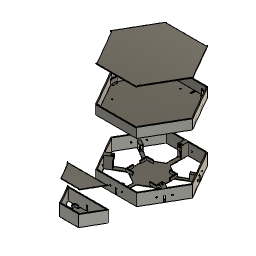
HiveLED (Autodesk Fusion 360 design; units mm, degrees)
Autodesk Fusion 360 part; units mm, degrees
sketch "Sketch1" plane through (0, 0, 0) normal (0, 0, 1) x (1, 0, 0) in component "base"
  line L0 (-43.3013, 75) -> (-86.6025, 0)
  line L1 (-86.6025, 0) -> (-43.3013, -75)
  line L2 (-43.3013, -75) -> (43.3013, -75)
  line L3 (43.3013, -75) -> (86.6025, 0)
  line L4 (86.6025, 0) -> (43.3013, 75)
  line L5 (43.3013, 75) -> (-43.3013, 75)
  line L6 (-84.2931, 0) -> (-42.1466, -73)
  line L7 (-42.1466, -73) -> (42.1466, -73)
  line L8 (42.1466, -73) -> (84.2931, 0)
  line L9 (84.2931, 0) -> (42.1466, 73)
  line L10 (42.1466, 73) -> (-42.1466, 73)
  line L11 (-42.1466, 73) -> (-84.2931, 0)
  dimension "d11" = 150
  dimension "d12" = -2
  constraint horizontal L3.end origin
  measures "d11" distance of L2 L5
extrude "Extrude11" add sketch "Sketch1" along normal blind 3 contours L0 L1 L2 L3 L4 L5 | L6 L7 L8 L9 L10 L11 makes body 1 in component "base"
extrude "Extrude12" add sketch "Sketch1" along normal blind 23 bodies 1 in component "base"
sketch "Sketch5" plane through (0, 0, 3) normal (0, 0, 1) x (-1, 0, 0)
  line L0 (84.2931, 0) -> (42.1466, 73)
  line L1 (42.1466, 73) -> (-42.1466, 73)
  line L2 (-42.1466, 73) -> (-84.2931, 0)
  line L3 (-84.2931, 0) -> (-42.1466, -73)
  line L4 (-42.1466, -73) -> (42.1466, -73)
  line L5 (42.1466, -73) -> (84.2931, 0)
  line L6 (79.53, -8.25) -> (79.53, 8.25)
  line L7 (46.9097, 64.75) -> (32.6203, 73)
  line L8 (-32.6203, 73) -> (-46.9097, 64.75)
  line L9 (-79.53, 8.25) -> (-79.53, -8.25)
  line L10 (-46.9097, -64.75) -> (-32.6203, -73)
  line L11 (32.6203, -73) -> (46.9097, -64.75)
  dimension "d82" = 16.5
  dimension "d84" = 360
  constraint coincident L5 L6.start
  constraint coincident L0 L6.end
  constraint vertical L6
  measures "d82" distance of L6.start L6.end
extrude "Extrude13" add sketch "Sketch5" along normal blind 10.1 contours L0 L5 L6 | L0 L1 L7 | L4 L5 L11 | L1 L2 L8 | L3 L4 L10 | L2 L3 L9 bodies 1 in component "base"
sketch "Sketch6" plane through (0, 0, 0) normal (0, 1, 0) x (1, 0, 0)
  line L0 (84.2931, -13.1) -> (84.2931, -23)
  line L1 (84.2931, -23) -> (86.6025, -23)
  line L2 (86.6025, -23) -> (86.6025, 0)
  line L3 (86.6025, 0) -> (-86.6025, 0)
  line L4 (-86.6025, 0) -> (-86.6025, -23)
  line L5 (-86.6025, -23) -> (-84.2931, -23)
  line L6 (-84.2931, -23) -> (-84.2931, -13.1)
  line L7 (-84.2931, -13.1) -> (-79.53, -13.1)
  line L8 (-79.53, -13.1) -> (-79.53, -3)
  line L9 (-79.53, -3) -> (79.53, -3)
  line L10 (79.53, -3) -> (79.53, -13.1)
  line L11 (79.53, -13.1) -> (84.2931, -13.1)
  line L12 (79.13, -3) -> (79.13, -5)
  line L13 (79.13, -5) -> (77.13, -3)
  dimension "d87" = 2
  dimension "d88" = 45
  dimension "d89" = 0.4
  constraint coincident L9 L12.start
  constraint perpendicular L9 L12
  constraint coincident L9 L13.end
  measures "d87" distance of L12.start L12.end
  measures "d88" angle of L12 L13
  measures "d89" distance of L10 L12
extrude "Extrude14" add sketch "Sketch6" along normal mid plane 10 contours L9 L12 L13 bodies 1 in component "base"
pattern_circular "C-Pattern3" count 6 over 360 about axis through (0, 0, 1.75) along (0, 0, 1) of "Extrude14" in component "base"
sketch "Sketch17" plane through (0, 0, 23) normal (0, 0, 1) x (-1, 0, 0) in component "base"
  line L0 (84.2931, 0) -> (42.1466, -73)
  line L1 (42.1466, -73) -> (-42.1466, -73)
  line L2 (-42.1466, -73) -> (-84.2931, 0)
  line L3 (-84.2931, 0) -> (-42.1466, 73)
  line L4 (-42.1466, 73) -> (42.1466, 73)
  line L5 (42.1466, 73) -> (84.2931, 0)
  line L6 (-43.3013, -75) -> (43.3013, -75)
  line L7 (43.3013, -75) -> (86.6025, 0)
  line L8 (86.6025, 0) -> (43.3013, 75)
  line L9 (43.3013, 75) -> (-43.3013, 75)
  line L10 (-43.3013, 75) -> (-86.6025, 0)
  line L11 (-86.6025, 0) -> (-43.3013, -75)
  line L12 (42.1466, 73) -> (43.3013, 75)
  line L13 (-43.3013, 75) -> (-42.1466, 73)
  line L14 (-42.1466, -73) -> (-43.3013, -75)
  line L15 (-84.2931, 0) -> (-86.6025, 0)
  line L16 (42.1466, -73) -> (43.3013, -75)
  line L17 (84.2931, 0) -> (86.6025, 0)
  constraint coincident L4.end L5.start
  constraint coincident L8.end L9.start
  constraint coincident L9.end L10.start
  constraint coincident L3.end L4.start
  constraint coincident L1.end L2.start
  constraint coincident L6.start L11.end
  constraint coincident L2.end L3.start
  constraint coincident L10.end L11.start
  constraint coincident L0.end L1.start
  constraint coincident L6.end L7.start
  constraint coincident L0.start L5.end
  constraint coincident L7.end L8.start
extrude "Extrude27" cut sketch "Sketch17" against normal blind 3 contours L0 L7 L16 L17 | L4 L9 L12 L13 | L2 L11 L14 L15 bodies 1 in component "base"
sketch "Sketch19" plane through (0, 0, 20) normal (0, 0, 1) x (-1, 0, 0) in component "base"
  line L0 (-43.3013, 75) -> (-42.1466, 73)
  line L1 (-42.1466, 73) -> (42.1466, 73)
  line L2 (42.1466, 73) -> (43.3013, 75)
  line L3 (43.3013, 75) -> (-43.3013, 75)
  line L4 (42.1466, -73) -> (43.3013, -75)
  line L5 (43.3013, -75) -> (86.6025, 0)
  line L6 (86.6025, 0) -> (84.2931, 0)
  line L7 (84.2931, 0) -> (42.1466, -73)
  line L8 (-42.1466, -73) -> (-84.2931, 0)
  line L9 (-84.2931, 0) -> (-86.6025, 0)
  line L10 (-86.6025, 0) -> (-43.3013, -75)
  line L11 (-43.3013, -75) -> (-42.1466, -73)
  line L12 (84.2931, 0) -> (42.1466, 73)
  line L13 (-42.1466, 73) -> (42.1466, 73)
  line L14 (-42.1466, 73) -> (-84.2931, 0)
  line L15 (-42.1466, -73) -> (42.1466, -73)
  constraint coincident L6.end L7.start
  constraint coincident L1.end L2.start
  constraint coincident L0.end L1.start
  constraint coincident L8.end L9.start
  constraint coincident L8.start L11.end
  constraint coincident L4.start L7.end
extrude "Extrude31" cut 1 faces at (14.4338, -25, 0) along direction (0, 0, 1) blind 1.3 on bodies 1 bodies 1 in component "base"
extrude "Extrude1" add sketch "Sketch19" along normal blind 3 separate body makes body 2 in component "Top"
sketch "Sketch23" plane through (0, 0, 3) normal (0, 0, 1) x (-1, 0, 0) in component "base"
  line L0 (-35.2349, 71.0286) -> (-34.2349, 69.2965)
  line L1 (-34.2349, 69.2965) -> (-42.8951, 64.2965)
  line L2 (-42.8951, 64.2965) -> (-43.8951, 66.0286)
  line L3 (-43.8951, 66.0286) -> (-35.2349, 71.0286)
  line L4 (43.8951, 66.0286) -> (42.8951, 64.2965)
  line L5 (42.8951, 64.2965) -> (34.2349, 69.2965)
  line L6 (34.2349, 69.2965) -> (35.2349, 71.0286)
  line L7 (35.2349, 71.0286) -> (43.8951, 66.0286)
  line L8 (79.13, -5) -> (77.13, -5)
  line L9 (77.13, -5) -> (77.13, 5)
  line L10 (77.13, 5) -> (79.13, 5)
  line L11 (79.13, 5) -> (79.13, -5)
  line L12 (35.2349, -71.0286) -> (34.2349, -69.2965)
  line L13 (34.2349, -69.2965) -> (42.8951, -64.2965)
  line L14 (42.8951, -64.2965) -> (43.8951, -66.0286)
  line L15 (43.8951, -66.0286) -> (35.2349, -71.0286)
  line L16 (-43.8951, -66.0286) -> (-42.8951, -64.2965)
  line L17 (-42.8951, -64.2965) -> (-34.2349, -69.2965)
  line L18 (-34.2349, -69.2965) -> (-35.2349, -71.0286)
  line L19 (-35.2349, -71.0286) -> (-43.8951, -66.0286)
  line L20 (-79.13, 5) -> (-77.13, 5)
  line L21 (-77.13, 5) -> (-77.13, -5)
  line L22 (-77.13, -5) -> (-79.13, -5)
  line L23 (-79.13, -5) -> (-79.13, 5)
  line L24 (46.9097, 64.75) -> (32.6203, 73)
  line L25 (32.6203, 73) -> (-32.6203, 73)
  line L26 (-32.6203, 73) -> (-46.9097, 64.75)
  line L27 (-46.9097, 64.75) -> (-79.53, 8.25)
  line L28 (-79.53, 8.25) -> (-79.53, -8.25)
  line L29 (-79.53, -8.25) -> (-46.9097, -64.75)
  line L30 (-46.9097, -64.75) -> (-32.6203, -73)
  line L31 (-32.6203, -73) -> (32.6203, -73)
  line L32 (32.6203, -73) -> (46.9097, -64.75)
  line L33 (46.9097, -64.75) -> (79.53, -8.25)
  line L34 (79.53, -8.25) -> (79.53, 8.25)
  line L35 (79.53, 8.25) -> (46.9097, 64.75)
  circle A0 centre (0, -61.45) radius 1.55
  point P0 (0, -61.45)
  dimension "d219" = 3.1
  dimension "d220" = 11.55
  constraint vertical origin A0.centre
  constraint coincident P0 A0.centre
  measures "d219" diameter of A0
  measures "d220" distance of L31 P0
extrude "Extrude38" cut sketch "Sketch23" against normal blind 1.7 contours A0 bodies 1 in component "base"
pattern_circular "C-Pattern5" count 3 over 360 about axis through (0, 0, 1.75) along (0, 0, 1) of "Extrude38" in component "base"
sketch "Sketch24" plane through (0, 0, 1.3) normal (0, 0, -1) x (1, 0, 0) in component "base"
  circle A0 centre (53.2173, 30.725) radius 1.55
  circle A1 centre (-53.2173, 30.725) radius 1.55
  circle A2 centre (0, -61.45) radius 1.55
  line L0 (-43.3013, -75) -> (43.3013, -75)
  line L1 (43.3013, -75) -> (86.6025, 0)
  line L2 (86.6025, 0) -> (43.3013, 75)
  line L3 (43.3013, 75) -> (-43.3013, 75)
  line L4 (-43.3013, 75) -> (-86.6025, 0)
  line L5 (-86.6025, 0) -> (-43.3013, -75)
  line L6 (-42.1466, -73) -> (42.1466, -73)
  line L7 (42.1466, -73) -> (84.2931, 0)
  line L8 (84.2931, 0) -> (42.1466, 73)
  line L9 (42.1466, 73) -> (-42.1466, 73)
  line L10 (-42.1466, 73) -> (-84.2931, 0)
  line L11 (-84.2931, 0) -> (-42.1466, -73)
  dimension "d230" = -2
extrude "Extrude1'" add sketch "Sketch24" along normal blind 25 separate body contours L0 L1 L2 L3 L4 L5 makes body 3 in component "Electronics Cabin"
sketch "Sketch1 (2)" plane through (64.9519, -37.5, 0) normal (0.866025, -0.5, 0) x (0.5, 0.866025, 0) in component "Electronics Cabin"
  line L0 (-43.3013, 1.3) -> (-43.3013, -23.7)
  line L1 (43.3013, -23.7) -> (43.3013, 1.3)
  line L2 (-1.5, -11.7) -> (1.5, -11.7)
  line L3 (1.5, -11.7) -> (1.5, -22.7)
  line L4 (1.5, -22.7) -> (-1.5, -22.7)
  line L5 (-1.5, -22.7) -> (-1.5, -11.7)
  line L6 (-1.5, -11.7) -> (1.5, -22.7) construction
  line L7 (1.5, -11.7) -> (-1.5, -22.7) construction
  line L8 (-42.1466, 1.3) -> (42.1466, 1.3) construction
  line L9 (42.1466, 1.3) -> (42.1466, -23.7) construction
  line L10 (42.1466, -23.7) -> (-42.1466, -23.7)
  line L11 (-42.1466, -23.7) -> (-42.1466, 1.3) construction
  line L12 (3, -24.2) -> (-3, -24.2)
  line L13 (-3, -24.2) -> (-3, -10.2)
  line L14 (-3, -10.2) -> (3, -10.2)
  line L15 (3, -10.2) -> (3, -24.2)
  point P0 (0, -17.2)
  dimension "d243" = 3
  dimension "d244" = 11
  dimension "d245" = 1
  dimension "d246" = -1.5
  constraint horizontal L2
  constraint perpendicular L2 L3
  constraint parallel L2 L4
  constraint parallel L3 L5
  constraint coincident L6 P0
  constraint coincident L7 P0
  constraint vertical origin P0
  measures "d243" distance of L3 L5
  measures "d244" distance of L2.end L3.end
  measures "d245" distance of L4 L10
extrude "Extrude2" add sketch "Sketch1 (2)" against normal blind 15.45 contours L10 L13 L14 L15 bodies 3 in component "Electronics Cabin"
extrude "Extrude4" cut sketch "Sketch1 (2)" against normal blind 2 contours L2 L3 L4 L5 bodies 3 in component "Electronics Cabin"
sketch "Sketch2" plane through (0, 0, -23.7) normal (0, 0, -1) x (1, 0, 0) in component "Electronics Cabin"
  line L0 (43.3013, 75) -> (-43.3013, 75)
  line L1 (-43.3013, 75) -> (-86.6025, 0)
  line L2 (-86.6025, 0) -> (-43.3013, -75)
  line L3 (-43.3013, -75) -> (43.3013, -75)
  line L4 (43.3013, -75) -> (86.6025, 0)
  line L5 (86.6025, 0) -> (43.3013, 75)
  line L6 (64.7199, 33.9019) -> (84.2931, 0)
  line L7 (84.2931, 0) -> (42.1466, -73)
  line L8 (42.1466, -73) -> (-42.1466, -73)
  line L9 (-42.1466, -73) -> (-84.2931, 0)
  line L10 (-84.2931, 0) -> (-42.1466, 73)
  line L11 (-42.1466, 73) -> (42.1466, 73)
  line L12 (61.7199, 39.0981) -> (50.0718, 32.3731)
  line L13 (53.0718, 27.1769) -> (64.7199, 33.9019)
  line L14 (42.1466, 73) -> (61.7199, 39.0981)
  line L15 (50.0718, 32.3731) -> (53.0718, 27.1769)
extrude "Extrude5" add sketch "Sketch2" against normal blind 1 contours L6 L7 L8 L9 L10 L11 L12 L13 L14 L15 bodies 3 in component "Electronics Cabin"
pattern_circular "C-Pattern1" count 6 over 360 about axis through (0, 0, 1.75) along (0, 0, 1) of "Extrude2", "Extrude4" in component "Electronics Cabin"
sketch "Sketch3" plane through (0, 0, 0) normal (1, 0, 0) x (0, 1, 0) in component "Electronics Cabin"
  line L0 (-75, -11.7) -> (-59.55, -11.7)
  line L1 (-59.55, -10.2) -> (-73, -10.2)
  line L2 (-73, -10.2) -> (-73, 1.3)
  line L3 (-73, 1.3) -> (-75, 1.3)
  line L4 (-75, 1.3) -> (-75, -11.7)
  line L5 (59.55, -11.7) -> (75, -11.7)
  line L6 (75, -11.7) -> (75, 1.3)
  line L7 (75, 1.3) -> (73, 1.3)
  line L8 (73, 1.3) -> (73, -10.2)
  line L9 (73, -10.2) -> (59.55, -10.2)
  line L10 (75, -22.7) -> (-75, -22.7)
  line L11 (-75, -22.7) -> (-75, -23.7)
  line L12 (-75, -23.7) -> (75, -23.7)
  line L13 (75, -23.7) -> (75, -22.7)
  line L14 (63, 3) -> (63, 1.3)
  line L15 (75, 1.3) -> (75, 23)
  line L16 (75, 23) -> (73, 23)
  line L17 (73, 23) -> (73, 3)
  line L18 (59.9, 1.3) -> (59.9, 3)
  line L19 (63, 1.3) -> (75, 1.3)
  line L20 (-73, 20) -> (-75, 20)
  line L21 (-75, 20) -> (-75, 1.3)
  line L22 (-75, 1.3) -> (59.9, 1.3)
  line L23 (73, 3) -> (63, 3)
  line L24 (59.9, 3) -> (-73, 3)
  line L25 (-73, 3) -> (-73, 20)
  line L26 (58.65, 1.3) -> (58.65, -3.6)
  line L27 (58.65, -0.2) -> (64.25, -0.2)
  line L28 (64.25, -0.2) -> (64.25, -2.6)
  line L29 (64.25, -2.6) -> (58.65, -2.6)
  line L30 (61.45, -0.2) -> (61.45, -2.6) construction
  line L31 (59.9, 3) -> (63, 3) construction
  line L32 (59.55, -10.2) -> (58.65, -3.6)
  line L33 (59.55, -10.2) -> (58.5867, -10.2117) construction
  line L34 (75, 1.3) -> (63, 1.3)
  line L35 (-59.55, -11.7) -> (-59.55, -10.2)
  line L36 (59.55, -10.2) -> (59.55, -11.7)
  line L37 (59.9, 1.3) -> (63, 1.3)
  point P0 (61.45, 3)
  dimension "d255" = 5.6
  dimension "d256" = 1.5
  dimension "d258" = 2.4
  dimension "d260" = 1
  constraint coincident L19 L26.start
  constraint perpendicular L19 L26
  constraint coincident L26 L27.start
  constraint perpendicular L26 L27
  constraint perpendicular L27 L28
  constraint coincident L26 L29.end
  constraint perpendicular L26 L29
  constraint midpoint L27 L30.start
  constraint midpoint L29 L30.end
  constraint coincident L18.end L24.start
  constraint coincident L14.start L23.end
  constraint midpoint L31 P0
  constraint vertical L30.start P0
  constraint coincident L9.end L32.start
  constraint coincident L6.end L7.start
  constraint coincident L14.end L19.start
  constraint coincident L18.start L22.end
  measures "d255" distance of L27.start L27.end
  measures "d256" distance of L19 L27
  measures "d258" distance of L27 L29
  measures "d260" distance of L26.end L29.end
extrude "Extrude6" add sketch "Sketch3" along normal mid plane 8.2 contours L8 L9 L19 L22 L26 L27 L28 L29 L32 L34 L37 bodies 3 in component "Electronics Cabin"
sketch "Sketch4" plane through (0, 58.65, 0) normal (0, -1, 0) x (1, 0, 0) in component "Electronics Cabin"
  line L0 (-4.1, -3.6) -> (4.1, -3.6)
  line L1 (4.1, -3.6) -> (4.1, -2.6)
  line L2 (4.1, -2.6) -> (-4.1, -2.6)
  line L3 (-4.1, -2.6) -> (-4.1, -3.6)
  line L4 (-4.1, -0.2) -> (4.1, -0.2)
  line L5 (4.1, -0.2) -> (4.1, 1.3)
  line L6 (-4.1, 1.3) -> (-4.1, -0.2)
  line L7 (-4.1, -0.2) -> (-2.8, -0.2)
  line L8 (-2.8, -0.2) -> (-2.8, -2.6)
  line L9 (-2.8, -2.6) -> (-4.1, -2.6)
  line L10 (-4.1, -2.6) -> (-4.1, -0.2)
  line L11 (4.1, -0.2) -> (2.8, -0.2)
  line L12 (2.8, -0.2) -> (2.8, -2.6)
  line L13 (2.8, -2.6) -> (4.1, -2.6)
  line L14 (4.1, -2.6) -> (4.1, -0.2)
  line L15 (4.1, 1.3) -> (-4.1, 1.3)
  dimension "d287" = 5.6
  constraint horizontal L7
  constraint vertical L8
  constraint horizontal L9
  constraint vertical L10
  constraint coincident L2 L8.end
  constraint coincident L4.start L6.end
  constraint horizontal L11
  constraint vertical L12
  constraint horizontal L13
  constraint vertical L14
  constraint coincident L2 L12.end
  constraint coincident L4.end L5.start
  constraint equal L7 L11
  measures "d287" distance of L8 L12
extrude "Extrude7" add sketch "Sketch4" against normal blind 5.6 contours L2 L4 L7 L8 L9 L10 | L2 L4 L11 L12 L13 L14 bodies 3 in component "Electronics Cabin"
sketch "Sketch5 (2)" plane through (0, 0, 1.3) normal (0, 0, 1) x (-1, 0, 0) in component "Electronics Cabin"
  line L0 (84.2931, 0) -> (42.1466, -73)
  line L1 (42.1466, -73) -> (4.1, -73)
  line L2 (-42.1466, -73) -> (-84.2931, 0)
  line L3 (-84.2931, 0) -> (-42.1466, 73)
  line L4 (-42.1466, 73) -> (42.1466, 73)
  line L5 (42.1466, 73) -> (84.2931, 0)
  line L6 (43.3013, -75) -> (86.6025, 0)
  line L7 (86.6025, 0) -> (43.3013, 75)
  line L8 (43.3013, 75) -> (-43.3013, 75)
  line L9 (-43.3013, 75) -> (-86.6025, 0)
  line L10 (-86.6025, 0) -> (-43.3013, -75)
  line L11 (-43.3013, -75) -> (43.3013, -75)
  circle A0 centre (0, -61.45) radius 1.55
  line L12 (4.1, -73) -> (4.1, -58.65)
  line L13 (4.1, -58.65) -> (-4.1, -58.65)
  line L14 (-4.1, -58.65) -> (-4.1, -73)
  line L15 (-4.1, -73) -> (-42.1466, -73)
extrude "Extrude9" cut sketch "Sketch5 (2)" against normal blind 9 contours A0 bodies 3 in component "Electronics Cabin"
sketch "Sketch6 (2)" plane through (0, 0, -0.2) normal (0, 0, -1) x (1, 0, 0) in component "Electronics Cabin"
  circle A0 centre (0, -61.45) radius 1.55
  line L0 (2.8, -58.65) -> (-2.8, -58.65)
  line L1 (-2.8, -64.25) -> (2.8, -64.25)
  circle A1 centre (0, -61.45) radius 1.55
  line L2 (2.8, -64.25) -> (2.8, -58.65)
  line L3 (-2.8, -58.65) -> (-2.8, -64.25)
extrude "Extrude10" add sketch "Sketch6 (2)" against normal blind 0.3 contours A0 A1 bodies 3 in component "Electronics Cabin"
extrude "Extrude14'" add 2 faces at (-3.3667, 68.5167, -10.2) (3.3667, 64.0333, -10.2) along direction (0, 0, -1) blind 12.7 on bodies 3 bodies 3 in component "Electronics Cabin"
pattern_circular "C-Pattern2" count 3 over 360 about axis through (0, 0, 1.75) along (0, 0, 1) of "Extrude6", "Extrude7", "Extrude9", "Extrude10", "Extrude14'" in component "Electronics Cabin"
sketch "Sketch9" plane through (0, 0, 3) normal (0, 0, 1) x (-1, 0, 0)
  line L0 (-35.2349, 71.0286) -> (-34.2349, 69.2965)
  line L1 (-34.2349, 69.2965) -> (-42.8951, 64.2965)
  line L2 (-42.8951, 64.2965) -> (-43.8951, 66.0286)
  line L3 (-43.8951, 66.0286) -> (-35.2349, 71.0286)
  line L4 (43.8951, 66.0286) -> (42.8951, 64.2965)
  line L5 (42.8951, 64.2965) -> (34.2349, 69.2965)
  line L6 (34.2349, 69.2965) -> (35.2349, 71.0286)
  line L7 (35.2349, 71.0286) -> (43.8951, 66.0286)
  line L8 (79.13, -5) -> (77.13, -5)
  line L9 (77.13, -5) -> (77.13, 5)
  line L10 (77.13, 5) -> (79.13, 5)
  line L11 (79.13, 5) -> (79.13, -5)
  line L12 (35.2349, -71.0286) -> (34.2349, -69.2965)
  line L13 (34.2349, -69.2965) -> (42.8951, -64.2965)
  line L14 (42.8951, -64.2965) -> (43.8951, -66.0286)
  line L15 (43.8951, -66.0286) -> (35.2349, -71.0286)
  line L16 (-43.8951, -66.0286) -> (-42.8951, -64.2965)
  line L17 (-42.8951, -64.2965) -> (-34.2349, -69.2965)
  line L18 (-34.2349, -69.2965) -> (-35.2349, -71.0286)
  line L19 (-35.2349, -71.0286) -> (-43.8951, -66.0286)
  line L20 (-79.13, 5) -> (-77.13, 5)
  line L21 (-77.13, 5) -> (-77.13, -5)
  line L22 (-77.13, -5) -> (-79.13, -5)
  line L23 (-79.13, -5) -> (-79.13, 5)
  line L24 (46.9097, 64.75) -> (32.6203, 73)
  line L25 (32.6203, 73) -> (-32.6203, 73)
  line L26 (-32.6203, 73) -> (-46.9097, 64.75)
  line L27 (-46.9097, 64.75) -> (-79.53, 8.25)
  line L28 (-79.53, 8.25) -> (-79.53, -8.25)
  line L29 (-79.53, -8.25) -> (-46.9097, -64.75)
  line L30 (-46.9097, -64.75) -> (-32.6203, -73)
  line L31 (-32.6203, -73) -> (32.6203, -73)
  line L32 (32.6203, -73) -> (46.9097, -64.75)
  line L33 (46.9097, -64.75) -> (79.53, -8.25)
  line L34 (79.53, -8.25) -> (79.53, 8.25)
  line L35 (79.53, 8.25) -> (46.9097, 64.75)
  line L36 (-17.6203, -63.5) -> (-20.6203, -63.5)
  line L37 (-20.6203, -63.5) -> (-20.6203, -71.5)
  line L38 (-20.6203, -71.5) -> (-17.6203, -71.5)
  line L39 (-17.6203, -71.5) -> (-17.6203, -63.5)
  line L40 (-17.6203, -63.5) -> (-20.6203, -71.5) construction
  line L41 (-20.6203, -63.5) -> (-17.6203, -71.5) construction
  circle A0 centre (-53.2173, 30.725) radius 1.55
  circle A1 centre (53.2173, 30.725) radius 1.55
  circle A2 centre (0, -61.45) radius 1.55
  point P0 (-19.1203, -67.5)
  dimension "d319" = 8
  dimension "d320" = 3
  dimension "d321" = 1.5
  dimension "d322" = 12
  constraint horizontal L36
  constraint perpendicular L36 L37
  constraint parallel L36 L38
  constraint parallel L37 L39
  constraint coincident L40 P0
  constraint coincident L41 P0
  measures "d319" distance of L36.end L37.end
  measures "d320" distance of L37.end L38.end
  measures "d321" distance of L31 L38
  measures "d322" distance of L30.end L37
extrude "Extrude40" cut sketch "Sketch9" against normal blind 1.7 contours L36 L37 L38 L39 bodies 1 in component "base"
extrude "Extrude41" cut 3 faces at (14.0489, 74.3333, 23) (-71.399, -25, 23) (57.3501, -49.3333, 23) along direction (0, 0, -1) blind 1.3 on bodies 1 bodies 1 in component "base"
sketch "Sketch7" plane through (0, 0, -23.7) normal (0, 0, -1) x (1, 0, 0) in component "Electronics Cabin"
  line L0 (43.3013, 75) -> (-43.3013, 75)
  line L1 (-43.3013, 75) -> (-86.6025, 0)
  line L2 (-86.6025, 0) -> (-43.3013, -75)
  line L3 (-43.3013, -75) -> (43.3013, -75)
  line L4 (43.3013, -75) -> (86.6025, 0)
  line L5 (86.6025, 0) -> (43.3013, 75)
  line L6 (52.3218, -28.476) -> (65.7019, -36.201)
  line L7 (65.7019, -36.201) -> (64.2019, -38.799)
  line L8 (64.2019, -38.799) -> (50.8218, -31.074)
  line L9 (53.0718, -27.1769) -> (52.3218, -28.476)
  line L10 (84.2931, 0) -> (64.7199, -33.9019)
  line L11 (42.1466, -73) -> (4.1, -73)
  line L12 (1.5, -59.55) -> (1.5, -75)
  line L13 (1.5, -75) -> (-1.5, -75)
  line L14 (-1.5, -75) -> (-1.5, -59.55)
  line L15 (4.1, -59.55) -> (1.5, -59.55)
  line L16 (-4.1, -73) -> (-42.1466, -73)
  line L17 (-42.1466, -73) -> (-61.7199, -39.0981)
  line L18 (-50.8218, -31.074) -> (-64.2019, -38.799)
  line L19 (-64.2019, -38.799) -> (-65.7019, -36.201)
  line L20 (-65.7019, -36.201) -> (-52.3218, -28.476)
  line L21 (-50.0718, -32.3731) -> (-50.8218, -31.074)
  line L22 (-64.7199, -33.9019) -> (-84.2931, 0)
  line L23 (-84.2931, 0) -> (-65.2699, 32.9493)
  line L24 (-52.3218, 28.476) -> (-65.7019, 36.201)
  line L25 (-65.7019, 36.201) -> (-64.2019, 38.799)
  line L26 (-64.2019, 38.799) -> (-50.8218, 31.074)
  line L27 (-53.6218, 26.2243) -> (-52.3218, 28.476)
  line L28 (-61.1699, 40.0507) -> (-42.1466, 73)
  line L29 (-42.1466, 73) -> (-3, 73)
  line L30 (-1.5, 59.55) -> (-1.5, 75)
  line L31 (-1.5, 75) -> (1.5, 75)
  line L32 (1.5, 75) -> (1.5, 59.55)
  line L33 (-3, 59.55) -> (-1.5, 59.55)
  line L34 (3, 73) -> (42.1466, 73)
  line L35 (42.1466, 73) -> (61.1699, 40.0507)
  line L36 (50.8218, 31.074) -> (64.2019, 38.799)
  line L37 (64.2019, 38.799) -> (65.7019, 36.201)
  line L38 (65.7019, 36.201) -> (52.3218, 28.476)
  line L39 (65.2699, 32.9493) -> (84.2931, 0)
  line L40 (49.5218, 33.3257) -> (50.8218, 31.074)
  line L41 (0, 37.5278) -> (-32.5, 18.7639)
  line L42 (-32.5, 18.7639) -> (-32.5, -18.7639)
  line L43 (-32.5, -18.7639) -> (0, -37.5278)
  line L44 (0, -37.5278) -> (32.5, -18.7639)
  line L45 (32.5, -18.7639) -> (32.5, 18.7639)
  line L46 (32.5, 18.7639) -> (0, 37.5278)
  line L47 (4.1, -73) -> (4.1, -59.55)
  line L48 (-1.5, -59.55) -> (-4.1, -59.55)
  line L49 (-4.1, -59.55) -> (-4.1, -73)
  line L50 (-65.2699, 32.9493) -> (-53.6218, 26.2243)
  line L51 (-49.5218, 33.3257) -> (-61.1699, 40.0507)
  line L52 (61.1699, 40.0507) -> (49.5218, 33.3257)
  line L53 (52.3218, 28.476) -> (53.6218, 26.2243)
  line L54 (53.6218, 26.2243) -> (65.2699, 32.9493)
  line L55 (64.7199, -33.9019) -> (53.0718, -27.1769)
  line L56 (50.8218, -31.074) -> (50.0718, -32.3731)
  line L57 (50.0718, -32.3731) -> (61.7199, -39.0981)
  line L58 (61.7199, -39.0981) -> (42.1466, -73)
  line L59 (-61.7199, -39.0981) -> (-50.0718, -32.3731)
  line L60 (-52.3218, -28.476) -> (-53.0718, -27.1769)
  line L61 (-53.0718, -27.1769) -> (-64.7199, -33.9019)
  line L62 (-50.8218, 31.074) -> (-49.5218, 33.3257)
  line L63 (-3, 73) -> (-3, 59.55)
  line L64 (1.5, 59.55) -> (3, 59.55)
  line L65 (3, 59.55) -> (3, 73)
  line L66 (-4.1, -59.55) -> (-4.1, -35.1606)
  line L67 (4.1, -59.55) -> (4.1, -35.1606)
  line L68 (53.6218, 26.2243) -> (32.5, 14.0296)
  line L69 (49.5218, 33.3257) -> (28.4, 21.131)
  line L70 (-49.5218, 33.3257) -> (-28.4, 21.131)
  line L71 (-53.6218, 26.2243) -> (-32.5, 14.0296)
  line L72 (-50.0718, -32.3731) -> (-29.5, -20.4959)
  line L73 (-53.0718, -27.1769) -> (-32.5, -15.2998)
  line L74 (50.0718, -32.3731) -> (29.5, -20.4959)
  line L75 (53.0718, -27.1769) -> (32.5, -15.2998)
  line L76 (3, 59.55) -> (3, 35.7957)
  line L77 (-3, 59.55) -> (-3, 35.7957)
  dimension "d288" = 65
  dimension "d361" = 360
  dimension "d363" = 360
  constraint vertical L41.start origin
  constraint coincident L48.end L49.start
  constraint coincident L43 L66.end
  constraint perpendicular L48 L66
  constraint coincident L15.start L47.end
  constraint coincident L44 L67.end
  constraint perpendicular L15 L67
  constraint coincident L21.start L59.end
  constraint coincident L43 L72.end
  constraint perpendicular L21 L72
  constraint coincident L60.end L61.start
  constraint coincident L42 L73.end
  constraint perpendicular L60 L73
  measures "d288" distance of L42 L45
extrude "Extrude12'" cut sketch "Sketch7" against normal blind 1 contours L34 L35 L46 L52 L65 L69 L76 | L28 L29 L41 L51 L63 L70 L77 | L10 L39 L45 L54 L55 L68 L75 | L22 L23 L42 L50 L61 L71 L73 | L11 L44 L47 L57 L58 L67 L74 | L16 L17 L43 L49 L59 L66 L72 bodies 3 in component "Electronics Cabin"
sketch "Sketch8" plane through (0, 0, -22.7) normal (0, 0, 1) x (-1, 0, 0) in component "Electronics Cabin"
  line L0 (-29.5, -20.4959) -> (-4.1, -35.1606)
  line L1 (4.1, -35.1606) -> (29.5, -20.4959)
  line L2 (32.5, -15.2998) -> (32.5, 14.0296)
  line L3 (28.4, 21.131) -> (3, 35.7957)
  line L4 (-3, 35.7957) -> (-28.4, 21.131)
  line L5 (-32.5, 14.0296) -> (-32.5, -15.2998)
  line L6 (30.5, -20.5) -> (-30.5, -20.5)
  line L7 (-30.5, -20.5) -> (-30.5, 20.5)
  line L8 (-30.5, 20.5) -> (30.5, 20.5)
  line L9 (30.5, 20.5) -> (30.5, -20.5)
  line L10 (30.5, -20.5) -> (-30.5, 20.5) construction
  line L11 (-30.5, -20.5) -> (30.5, 20.5) construction
  line L12 (-32.5, 22.5) -> (32.5, 22.5)
  line L13 (32.5, 22.5) -> (32.5, -22.5)
  line L14 (32.5, -22.5) -> (-32.5, -22.5)
  line L15 (-32.5, -22.5) -> (-32.5, 22.5)
  line L16 (17.5, -22.5) -> (17.5, -20.5)
  line L17 (32.5, -7.5) -> (30.5, -7.5)
  line L18 (-20, 0) -> (-2.5, 0)
  line L19 (32.5, 7.5) -> (30.5, 7.5)
  line L20 (17.5, 22.5) -> (17.5, 20.5)
  line L21 (0, -2.5) -> (0, -20)
  line L22 (-17.5, -22.5) -> (-17.5, -20.5)
  line L23 (-32.5, -7.5) -> (-30.5, -7.5)
  line L24 (-32.5, 7.5) -> (-30.5, 7.5)
  line L25 (-17.5, 22.5) -> (-17.5, 20.5)
  line L26 (-32.5, 14.0296) -> (-32.5, -15.2998)
  line L27 (-29.5, -20.4959) -> (-4.1, -35.1606)
  line L28 (4.1, -35.1606) -> (29.5, -20.4959)
  line L29 (32.5, -15.2998) -> (32.5, 14.0296)
  line L30 (28.4, 21.131) -> (3, 35.7957)
  line L31 (-3, 35.7957) -> (-28.4, 21.131)
  line L32 (-4.1, -35.1606) -> (-4.1, -59.55)
  line L33 (-4.1, -59.55) -> (-1.5, -59.55)
  line L34 (-1.5, -59.55) -> (-1.5, -75)
  line L35 (-1.5, -75) -> (1.5, -75)
  line L36 (4.1, -59.55) -> (4.1, -35.1606)
  line L37 (-28.4, 21.131) -> (-49.5218, 33.3257)
  line L38 (53.6218, 26.2243) -> (52.3218, 28.476)
  line L39 (52.3218, 28.476) -> (65.7019, 36.201)
  line L40 (65.7019, 36.201) -> (64.2019, 38.799)
  line L41 (-53.6218, 26.2243) -> (-32.5, 14.0296)
  line L42 (-50.8218, 31.074) -> (-64.2019, 38.799)
  line L43 (-64.2019, 38.799) -> (-65.7019, 36.201)
  line L44 (-4.1, -35.1606) -> (-4.1, -59.55)
  line L45 (-4.1, -59.55) -> (-1.5, -59.55)
  line L46 (-1.5, -59.55) -> (-1.5, -75)
  line L47 (-1.5, -75) -> (1.5, -75)
  line L48 (4.1, -59.55) -> (4.1, -35.1606)
  line L49 (-28.4, 21.131) -> (-49.5218, 33.3257)
  line L50 (53.6218, 26.2243) -> (52.3218, 28.476)
  line L51 (52.3218, 28.476) -> (65.7019, 36.201)
  line L52 (65.7019, 36.201) -> (64.2019, 38.799)
  line L53 (-53.6218, 26.2243) -> (-32.5, 14.0296)
  line L54 (-50.8218, 31.074) -> (-64.2019, 38.799)
  line L55 (-64.2019, 38.799) -> (-65.7019, 36.201)
  line L56 (-32.5, -15.2998) -> (-53.0718, -27.1769)
  line L57 (-53.0718, -27.1769) -> (-52.3218, -28.476)
  line L58 (-52.3218, -28.476) -> (-65.7019, -36.201)
  line L59 (-65.7019, -36.201) -> (-64.2019, -38.799)
  line L60 (-64.2019, -38.799) -> (-50.8218, -31.074)
  line L61 (-50.8218, -31.074) -> (-50.0718, -32.3731)
  line L62 (-50.0718, -32.3731) -> (-29.5, -20.4959)
  line L63 (1.5, -75) -> (1.5, -59.55)
  line L64 (1.5, -59.55) -> (4.1, -59.55)
  line L65 (29.5, -20.4959) -> (50.0718, -32.3731)
  line L66 (50.0718, -32.3731) -> (50.8218, -31.074)
  line L67 (50.8218, -31.074) -> (64.2019, -38.799)
  line L68 (64.2019, -38.799) -> (65.7019, -36.201)
  line L69 (65.7019, -36.201) -> (52.3218, -28.476)
  line L70 (52.3218, -28.476) -> (53.0718, -27.1769)
  line L71 (53.0718, -27.1769) -> (32.5, -15.2998)
  line L72 (32.5, 14.0296) -> (53.6218, 26.2243)
  line L73 (64.2019, 38.799) -> (50.8218, 31.074)
  line L74 (50.8218, 31.074) -> (49.5218, 33.3257)
  line L75 (49.5218, 33.3257) -> (28.4, 21.131)
  line L76 (3, 35.7957) -> (3, 59.55)
  line L77 (3, 59.55) -> (1.5, 59.55)
  line L78 (1.5, 59.55) -> (1.5, 75)
  line L79 (1.5, 75) -> (-1.5, 75)
  line L80 (-1.5, 75) -> (-1.5, 59.55)
  line L81 (-1.5, 59.55) -> (-3, 59.55)
  line L82 (-3, 59.55) -> (-3, 35.7957)
  line L83 (-49.5218, 33.3257) -> (-50.8218, 31.074)
  line L84 (-65.7019, 36.201) -> (-52.3218, 28.476)
  line L85 (-52.3218, 28.476) -> (-53.6218, 26.2243)
  line L86 (-32.5, -15.2998) -> (-53.0718, -27.1769)
  line L87 (-53.0718, -27.1769) -> (-52.3218, -28.476)
  line L88 (-52.3218, -28.476) -> (-65.7019, -36.201)
  line L89 (-65.7019, -36.201) -> (-64.2019, -38.799)
  line L90 (-64.2019, -38.799) -> (-50.8218, -31.074)
  line L91 (-50.8218, -31.074) -> (-50.0718, -32.3731)
  line L92 (-50.0718, -32.3731) -> (-29.5, -20.4959)
  line L93 (1.5, -75) -> (1.5, -59.55)
  line L94 (1.5, -59.55) -> (4.1, -59.55)
  line L95 (29.5, -20.4959) -> (50.0718, -32.3731)
  line L96 (50.0718, -32.3731) -> (50.8218, -31.074)
  line L97 (50.8218, -31.074) -> (64.2019, -38.799)
  line L98 (64.2019, -38.799) -> (65.7019, -36.201)
  line L99 (65.7019, -36.201) -> (52.3218, -28.476)
  line L100 (52.3218, -28.476) -> (53.0718, -27.1769)
  line L101 (53.0718, -27.1769) -> (32.5, -15.2998)
  line L102 (32.5, 14.0296) -> (53.6218, 26.2243)
  line L103 (64.2019, 38.799) -> (50.8218, 31.074)
  line L104 (50.8218, 31.074) -> (49.5218, 33.3257)
  line L105 (49.5218, 33.3257) -> (28.4, 21.131)
  line L106 (3, 35.7957) -> (3, 59.55)
  line L107 (3, 59.55) -> (1.5, 59.55)
  line L108 (1.5, 59.55) -> (1.5, 75)
  line L109 (1.5, 75) -> (-1.5, 75)
  line L110 (-1.5, 75) -> (-1.5, 59.55)
  line L111 (-1.5, 59.55) -> (-3, 59.55)
  line L112 (-3, 59.55) -> (-3, 35.7957)
  line L113 (-49.5218, 33.3257) -> (-50.8218, 31.074)
  line L114 (-65.7019, 36.201) -> (-52.3218, 28.476)
  line L115 (-52.3218, 28.476) -> (-53.6218, 26.2243)
  dimension "d293" = 61
  dimension "d294" = 41
  dimension "d295" = -2
  dimension "d298" = 15
  dimension "d299" = 15
  constraint horizontal L6
  constraint perpendicular L6 L7
  constraint parallel L6 L8
  constraint parallel L7 L9
  constraint coincident L10 origin
  constraint coincident L11 origin
  constraint coincident L14 L16.start
  constraint coincident L6 L16.end
  constraint perpendicular L6 L16
  constraint coincident L2 L17.start
  constraint coincident L9 L17.end
  constraint perpendicular L9 L17
  constraint symmetric L16.start L18 L20.start
  constraint symmetric L16.end L18 L20.end
  constraint symmetric L17.start L18 L19.start
  constraint symmetric L17.end L18 L19.end
  constraint symmetric L16.start L21 L22.start
  constraint symmetric L16.end L21 L22.end
  constraint symmetric L17.start L21 L23.start
  constraint symmetric L17.end L21 L23.end
  constraint symmetric L19.start L21 L24.start
  constraint symmetric L19.end L21 L24.end
  constraint symmetric L20.start L21 L25.start
  constraint symmetric L20.end L21 L25.end
  measures "d293" distance of L7.end L8.end
  measures "d294" distance of L6.end L7.end
  measures "d298" distance of L13 L16
  measures "d299" distance of L14 L17
extrude "Extrude13'" add sketch "Sketch8" along normal blind 5 contours L0 L6 L14 L22 L27 | L0 L6 L14 L15 L27 L62 L92 | L5 L6 L7 L15 L23 L26 L62 L92 | L1 L6 L14 L16 L28 | L1 L6 L13 L14 L28 L65 L95 | L4 L5 L7 L8 L12 L15 L24 L25 L26 L31 L37 L49 | L2 L6 L9 L13 L17 L29 L65 L95 | L2 L3 L8 L9 L12 L13 L19 L20 L29 L30 L75 L105 | L4 L12 L31 L37 L49 | L3 L12 L30 L75 L105 bodies 3 in component "Electronics Cabin"
extrude "Extrude15" add 4 faces at (29.3406, 21.8333, -22.7) (-29.3406, 21.8333, -22.7) (-28.4, -22.0437, -22.7) (28.4, -22.0437, -22.7) along direction (0, 0, -1) blind 1 on bodies 3 bodies 3 in component "Electronics Cabin"
extrude "Extrude2'" cut 1 faces at (14.0489, -24.3333, 23) along direction (0, 0, -1) blind 1.3 on bodies 2 bodies 2 in component "Top"
extrude "Extrude42" add 6 faces at (-40.5589, 70.25, 13.1) (40.5589, 70.25, 13.1) (81.1177, 0, 13.1) (40.5589, -70.25, 13.1) (-40.5589, -70.25, 13.1) (-81.1177, 0, 13.1) along direction (0, 0, 1) blind 1 on bodies 1 bodies 1 in component "base"
sketch "Sketch26" plane through (0, 0, 14.1) normal (0, 0, 1) x (-1, 0, 0) in component "base"
  line L0 (42.1466, -73) -> (46.9097, -64.75)
  line L1 (46.9097, -64.75) -> (32.6203, -73)
  line L2 (32.6203, -73) -> (42.1466, -73)
  line L3 (45.9097, -66.4821) -> (34.6203, -73)
  line L4 (46.6499, -64.9) -> (56.8868, -47.1692)
  line L5 (56.8868, -47.1692) -> (12.4064, -72.85)
  line L6 (12.4064, -72.85) -> (32.8801, -72.85)
  line L7 (42.1466, -73) -> (84.2931, 0)
  line L8 (45.6499, -66.6321) -> (42.06, -72.85)
  line L9 (42.06, -72.85) -> (34.8801, -72.85)
  line L10 (34.8801, -72.85) -> (32.8801, -72.85)
  line L11 (45.6499, -66.6321) -> (46.6499, -64.9)
  dimension "d364" = 1
  dimension "d365" = 0.15
  dimension "d366" = 0.15
  dimension "d367" = 15
  dimension "d368" = 0.15
  dimension "d369" = 0.15
  constraint coincident L0 L3.start
  constraint coincident L2 L3.end
  constraint parallel L1 L3
  constraint coincident L1 L4.start
  constraint coincident L1 L6.end
  constraint horizontal L6
  constraint parallel L4 L7
  constraint parallel L1 L5
  constraint coincident L3 L8.start
  constraint coincident L3 L9.end
  constraint horizontal L9
  constraint parallel L7 L8
  measures "d364" distance of L1 L3
  measures "d365" distance of L4 L7
  measures "d366" distance of L2 L6
  measures "d367" distance of L0.start L5
  measures "d368" distance of L0 L8
  measures "d369" distance of L2 L9
extrude "Extrude43" cut sketch "Sketch26" against normal blind 2 contours L0 L2 L3 L7 L8 L9 | L3 L8 L9 bodies 1 in component "base"
pattern_circular "C-Pattern6" count 6 over 360 about axis through (0, 0, 1.75) along (0, 0, 1) of "Extrude43" in component "base"
extrude "Extrude44" add sketch "Sketch26" against normal blind 2 separate body contours L3 L8 L9 makes body 4 in component "base"
extrude "Extrude45" add sketch "Sketch26" along normal blind 1 separate body contours L3 L8 L9 | L1 L3 L10 L11 | L1 L4 L5 L6 makes body 5 in component "base"
combine "Combine4" operation add target body 5 tool bodies 4 in component "base"
sketch "Sketch1 (3)" plane through (0, 0, -23.7) normal (0, 0, -1) x (1, 0, 0) in component "Controller"
  line L0 (84.2931, 0) -> (64.7199, -33.9019)
  line L1 (32.5, -15.2998) -> (32.5, 14.0296)
  line L2 (61.1699, 40.0507) -> (30.7711, 22.5)
  line L3 (-32.5, 14.0296) -> (-32.5, -15.2998)
  line L4 (-64.7199, -33.9019) -> (-84.2931, 0)
  line L5 (-84.2931, 0) -> (-65.2699, 32.9493)
  line L6 (65.2699, 32.9493) -> (84.2931, 0)
  line L7 (26.0289, 22.5) -> (3, 35.7957)
  line L8 (3, 73) -> (42.1466, 73)
  line L9 (42.1466, -73) -> (4.1, -73)
  line L10 (4.1, -73) -> (4.1, -35.1606)
  line L11 (4.1, -35.1606) -> (26.0289, -22.5)
  line L12 (26.0289, -22.5) -> (32.5, -22.5)
  line L13 (-29.5, -20.4959) -> (-29.493, -20.5)
  line L14 (-4.1, -35.1606) -> (-4.1, -73)
  line L15 (-3, 35.7957) -> (-26.0289, 22.5)
  line L16 (32.5, 14.0296) -> (65.2699, 32.9493)
  line L17 (43.3013, 75) -> (-43.3013, 75)
  line L18 (-43.3013, 75) -> (-86.6025, 0)
  line L19 (-86.6025, 0) -> (-43.3013, -75)
  line L20 (-43.3013, -75) -> (43.3013, -75)
  line L21 (43.3013, -75) -> (86.6025, 0)
  line L22 (86.6025, 0) -> (43.3013, 75)
  line L23 (-43.3013, 75) -> (-20.2073, 115)
  line L24 (-20.2073, 115) -> (20.2073, 115)
  line L25 (43.3013, 75) -> (20.2073, 115)
  line L26 (-43.3013, 75) -> (43.3013, 75)
  line L27 (20.5, 108) -> (-20.5, 108)
  line L28 (-20.5, 108) -> (-20.5, 82)
  line L29 (-20.5, 82) -> (20.5, 82)
  line L30 (20.5, 82) -> (20.5, 108)
  line L31 (20.5, 108) -> (-20.5, 82) construction
  line L32 (-20.5, 108) -> (20.5, 82) construction
  line L33 (-29.4449, 95) -> (29.4449, 95) construction
  line L34 (-22.5, 80) -> (22.5, 80)
  line L35 (22.5, 80) -> (22.5, 110)
  line L36 (22.5, 110) -> (-22.5, 110)
  line L37 (-22.5, 110) -> (-22.5, 80)
  line L38 (-22.5, 102) -> (-20.5, 102)
  line L39 (-14.5, 108) -> (-14.5, 113)
  line L40 (-14.5, 82) -> (-14.5, 77)
  line L41 (-22.5, 88) -> (-20.5, 88)
  line L42 (0, 82) -> (0, 108) construction
  line L43 (14.5, 108) -> (14.5, 113)
  line L44 (22.5, 102) -> (20.5, 102)
  line L45 (22.5, 88) -> (20.5, 88)
  line L46 (14.5, 82) -> (14.5, 77)
  line L47 (-22.5, 88) -> (-33.4863, 88)
  line L48 (-22.5, 102) -> (-25.4034, 102)
  line L49 (22.5, 102) -> (25.4034, 102)
  line L50 (22.5, 88) -> (33.4863, 88)
  line L51 (3, 35.7957) -> (3, 73)
  line L52 (-32.5, -15.2998) -> (-64.7199, -33.9019)
  line L53 (29.5, -20.4959) -> (29.507, -20.5)
  line L54 (-29.493, -20.5) -> (-29.507, -20.5)
  line L55 (29.493, -20.5) -> (29.5, -20.4959)
  line L56 (-29.507, -20.5) -> (-29.5, -20.4959)
  line L57 (29.507, -20.5) -> (29.493, -20.5)
  line L58 (64.7199, -33.9019) -> (32.5, -15.2998)
  line L59 (-65.2699, 32.9493) -> (-32.5, 14.0296)
  line L60 (30.7711, 22.5) -> (26.0289, 22.5)
  line L61 (42.1466, 73) -> (61.1699, 40.0507)
  line L62 (32.5, -22.5) -> (32.5, -22.228)
  line L63 (32.5, -22.228) -> (61.7199, -39.0981)
  line L64 (61.7199, -39.0981) -> (42.1466, -73)
  line L65 (-32.5, -22.228) -> (-32.5, -22.5)
  line L66 (-32.5, -22.5) -> (-26.0289, -22.5)
  line L67 (-26.0289, -22.5) -> (-4.1, -35.1606)
  line L68 (-4.1, -73) -> (-42.1466, -73)
  line L69 (-42.1466, -73) -> (-61.7199, -39.0981)
  line L70 (-61.7199, -39.0981) -> (-32.5, -22.228)
  line L71 (-3, 73) -> (-3, 35.7957)
  line L72 (-26.0289, 22.5) -> (-30.7711, 22.5)
  line L73 (-30.7711, 22.5) -> (-61.1699, 40.0507)
  line L74 (-61.1699, 40.0507) -> (-42.1466, 73)
  line L75 (-42.1466, 73) -> (-3, 73)
  line L76 (-39.8372, 77) -> (39.8372, 77)
  line L77 (39.8372, 77) -> (19.0526, 113)
  line L78 (-19.0526, 113) -> (19.0526, 113)
  line L79 (-39.8372, 77) -> (-19.0526, 113)
  point P0 (0, 95)
  dimension "d324" = 40
  dimension "d325" = -2
  dimension "d326" = 41
  dimension "d327" = 26
  dimension "d328" = 2
  dimension "d329" = 6
  dimension "d330" = 6
  constraint coincident L17.end L18.start
  constraint parallel L18 L23
  constraint parallel L17 L24
  constraint coincident L17.start L22.end
  constraint parallel L22 L25
  constraint horizontal L27
  constraint perpendicular L27 L28
  constraint parallel L27 L29
  constraint parallel L28 L30
  constraint coincident L31 P0
  constraint coincident L32 P0
  constraint vertical origin P0
  constraint midpoint L33.start L79
  constraint midpoint L33.end L77
  constraint coincident P0 L33
  constraint coincident L37 L38.start
  constraint coincident L28 L38.end
  constraint perpendicular L28 L38
  constraint coincident L27 L39.start
  constraint symmetric L33 L38.start L41.start
  constraint symmetric L33 L38.end L41.end
  constraint symmetric L33 L39.start L40.start
  constraint symmetric L33 L39.end L40.end
  constraint midpoint L29 L42.start
  constraint midpoint L27 L42.end
  constraint symmetric L38.start L42 L44.start
  constraint symmetric L38.end L42 L44.end
  constraint symmetric L39.start L42 L43.start
  constraint symmetric L39.end L42 L43.end
  constraint symmetric L40.start L42 L46.start
  constraint symmetric L40.end L42 L46.end
  constraint symmetric L41.start L42 L45.start
  constraint symmetric L41.end L42 L45.end
  constraint coincident L47.end L79
  constraint perpendicular L37 L47
  constraint coincident L48.end L79
  constraint perpendicular L37 L48
  constraint coincident L49.end L77
  constraint perpendicular L35 L49
  constraint coincident L50.end L77
  constraint perpendicular L35 L50
  measures "d324" distance of L17 L24
  measures "d326" distance of L28.end L29.end
  measures "d327" distance of L27.end L28.end
  measures "d329" distance of L27 L38
  measures "d330" distance of L28 L39
extrude "Extrude4'" add sketch "Sketch1 (3)" against normal blind 25 separate body contours L17 L23 L24 L25 L26 | L35 L36 L77 | L36 L37 L79 makes body 6 in component "Controller"
extrude "Extrude5'" add sketch "Sketch1 (3)" against normal blind 1 contours L27 L28 L29 L30 | L27 L30 L35 L36 L43 L44 L77 | L27 L36 L39 L43 | L30 L35 L44 L45 | L27 L28 L36 L37 L38 L39 L79 | L36 L39 L43 L78 | L29 L30 L34 L35 L45 L46 | L35 L49 L50 L77 | L28 L37 L38 L41 | L29 L34 L40 L46 | L28 L29 L34 L37 L40 L41 | L37 L47 L48 L79 | L34 L40 L46 L76 bodies 6 in component "Controller"
extrude "Extrude6'" add sketch "Sketch1 (3)" against normal blind 6 contours L27 L30 L35 L36 L43 L44 L77 | L27 L28 L36 L37 L38 L39 L79 | L29 L30 L34 L35 L45 L46 | L35 L36 L77 | L36 L37 L79 | L28 L29 L34 L37 L40 L41 bodies 6 in component "Controller"
sketch "Sketch2 (2)" plane through (0, -77, 0) normal (0, -1, 0) x (1, 0, 0) in component "Controller"
  line L0 (14.5, -22.7) -> (14.5, -23.7)
  line L1 (14.5, -23.7) -> (39.8372, -23.7)
  line L2 (39.8372, -23.7) -> (39.8372, 1.3)
  line L3 (39.8372, 1.3) -> (-39.8372, 1.3)
  line L4 (-39.8372, 1.3) -> (-39.8372, -23.7)
  line L5 (-14.5, -22.7) -> (14.5, -22.7)
  line L6 (1.5, -22.7) -> (1.5, -11.7)
  line L7 (1.5, -11.7) -> (-1.5, -11.7)
  line L8 (-1.5, -11.7) -> (-1.5, -22.7)
  line L9 (1.5, -22.7) -> (-1.5, -22.7)
  line L10 (-39.8372, -23.7) -> (-14.5, -23.7)
  line L11 (-14.5, -23.7) -> (-14.5, -22.7)
extrude "Extrude7'" cut sketch "Sketch2 (2)" against normal blind 2 contours L5 L6 L7 L8 L9 bodies 6 in component "Controller"
sketch "Sketch3 (2)" plane through (0, 0, 1.3) normal (0, 0, 1) x (-1, 0, 0) in component "Controller"
  line L0 (-39.8372, 77) -> (-19.0526, 113)
  line L1 (19.0526, 113) -> (39.8372, 77)
  line L2 (39.8372, 77) -> (-39.8372, 77)
  line L3 (43.3013, 75) -> (20.2073, 115)
  line L4 (-20.2073, 115) -> (-43.3013, 75)
  line L5 (-43.3013, 75) -> (43.3013, 75)
  line L6 (39.8372, 77) -> (43.3013, 75)
  line L7 (19.0526, 113) -> (20.2073, 115)
  line L8 (-19.0526, 113) -> (-20.2073, 115)
  line L9 (-39.8372, 77) -> (-43.3013, 75)
  line L10 (-19.0526, 113) -> (19.0526, 113)
  line L11 (20.2073, 115) -> (-20.2073, 115)
  constraint coincident L1.end L2.start
  constraint coincident L3.start L5.end
  constraint coincident L1.start L7.start
  constraint coincident L3.end L7.end
  constraint coincident L0.end L8.start
  constraint coincident L4.start L8.end
  constraint coincident L0.start L2.end
  constraint coincident L4.end L5.start
extrude "Extrude8" cut sketch "Sketch3 (2)" against normal blind 1 contours L0 L4 L8 L9 | L1 L3 L6 L7 bodies 6 in component "Controller"
sketch "Sketch4 (2)" plane through (0, 0, 0.3) normal (0, 0, 1) x (-1, 0, 0) in component "Controller"
  line L0 (39.8372, 77) -> (43.3013, 75)
  line L1 (43.3013, 75) -> (20.2073, 115)
  line L2 (19.0526, 113) -> (39.8372, 77)
  line L3 (-20.2073, 115) -> (-43.3013, 75)
  line L4 (-43.3013, 75) -> (-39.8372, 77)
  line L5 (-39.8372, 77) -> (-19.0526, 113)
  line L6 (43.3013, 75) -> (39.8372, 77)
  line L7 (39.8372, 77) -> (-39.8372, 77)
  line L8 (-39.8372, 77) -> (-43.3013, 75)
  line L9 (-43.3013, 75) -> (43.3013, 75)
  line L10 (39.8372, 77) -> (14.3435, 105.7098)
  line L11 (15.8404, 106.9806) -> (43.3013, 75)
  line L12 (20.2073, 115) -> (19.0526, 113)
  line L13 (-19.0526, 113) -> (-20.2073, 115)
  line L14 (19.0526, 113) -> (20.2073, 115)
  line L15 (20.2073, 115) -> (-20.2073, 115)
  line L16 (-20.2073, 115) -> (-19.0526, 113)
  line L17 (-19.0526, 113) -> (19.0526, 113)
  constraint coincident L0.start L2.end
  constraint coincident L0.end L1.start
extrude "Extrude9'" add sketch "Sketch4 (2)" along normal blind 1 separate body contours L0 L2 L6 L11 | L2 L5 L7 L17 | L3 L4 L5 L8 L13 L16 makes body 7 in component "Controller"
sketch "Sketch9 (2)" plane through (0, -73, 0) normal (0, 1, 0) x (-1, 0, 0) in component "Electronics Cabin"
  line L0 (42.1466, 1.3) -> (-42.1466, 1.3)
  line L1 (-42.1466, 1.3) -> (-42.1466, -23.7)
  line L2 (3, -23.7) -> (42.1466, -23.7)
  circle A0 centre (12.2687, -12.2877) radius 1.55
  line L3 (0, 1.3) -> (22.5733, -23.7) construction
  line L4 (-42.1466, -11.2) -> (-3.9234, -11.964) construction
  line L5 (0, 20) -> (0, 2.5) construction
  circle A1 centre (-12.2687, -12.2877) radius 1.55
  line L6 (3, -10.2) -> (3, -23.7)
  line L7 (42.1466, -23.7) -> (42.1466, 1.3)
  line L8 (-3, -23.7) -> (-3, -10.2)
  line L9 (-3, -10.2) -> (3, -10.2)
  line L10 (-42.1466, -23.7) -> (-3, -23.7)
  dimension "d352" = 3.1
  constraint midpoint L0 L3.start
  constraint midpoint L2 L3.end
  constraint midpoint L1 L4.start
  constraint coincident A0.centre L4
  constraint coincident A0.centre L3
  constraint symmetric A0 L5 A1
  measures "d352" diameter of A0
extrude "Extrude16" cut sketch "Sketch9 (2)" against normal blind 2 contours A0 | A1 bodies 3 in component "Electronics Cabin"
pattern_circular "C-Pattern3'" count 6 over 360 about axis through (0, 0, 1.75) along (0, 0, 1) of "Extrude16" in component "Electronics Cabin"
move_face "OffsetFaces4" offset -0.15 2 faces at (40.9919, -76.3333, 0.9667) (-42.1466, -75.6667, 0.9667) on bodies 7 in component "Controller"
sketch "Sketch5 (3)" plane through (0, -77, 0) normal (0, -1, 0) x (1, 0, 0) in component "Controller"
  line L0 (1.5, -11.7) -> (1.5, -22.7)
  line L1 (1.5, -22.7) -> (14.5, -22.7)
  line L2 (14.5, -22.7) -> (14.5, -23.7)
  line L3 (14.5, -23.7) -> (39.8372, -23.7)
  line L4 (39.8372, -23.7) -> (39.8372, 0.3)
  line L5 (39.8372, 0.3) -> (39.8372, 1.3)
  line L6 (39.8372, 1.3) -> (-39.8372, 1.3)
  line L7 (-39.8372, 1.3) -> (-39.8372, 0.3)
  line L8 (-39.8372, 0.3) -> (-39.8372, -23.7)
  line L9 (-39.8372, -23.7) -> (-14.5, -23.7)
  line L10 (-14.5, -23.7) -> (-14.5, -22.7)
  line L11 (-14.5, -22.7) -> (-1.5, -22.7)
  line L12 (-1.5, -22.7) -> (-1.5, -11.7)
  line L13 (-1.5, -11.7) -> (1.5, -11.7)
  circle A0 centre (12.2687, -12.2877) radius 1.55
  circle A1 centre (-12.2687, -12.2877) radius 1.55
move_body "Move1" bodies 1 to x (1, 0, 0) y (0, 1, 0) z (0, 0, 1) at (0, 0, 100) in component "base"
move_body "Move1'" bodies 2 to x (1, 0, 0) y (0, 1, 0) z (0, 0, 1) at (0, 0, 175) in component "Top"
move_body "Move1''" bodies 6 to x (1, 0, 0) y (0, 1, 0) z (0, 0, 1) at (0, -60, 0) in component "Controller"
move_body "Move2" bodies 7 to x (1, 0, 0) y (0, 1, 0) z (0, 0, 1) at (0, -60, 45) in component "Controller"
extrude "Extrude10'" [suppressed] in component "Controller"
component "base" placed x (1, 0, 0) y (0, 1, 0) z (0, 0, 1) at (0, 0, 0)
component "Top" placed x (1, 0, 0) y (0, 1, 0) z (0, 0, 1) at (0, 0, 0) in component "base"
component "Electronics Cabin" placed x (1, 0, 0) y (0, 1, 0) z (0, 0, 1) at (0, 0, 0) in component "base"
component "Controller" placed x (1, 0, 0) y (0, 1, 0) z (0, 0, 1) at (0, 0, 0) in component "base"
equation "d220 = 10.00 mm + ( ( 3.1 / 2 ) * 1 mm )"
equation "d236 = -14.15 mm - 1.3 mm"
equation "d280 = -( 3 mm - 1.7 mm )"
named bodies: "Hex", "top", "Electronics Cabin", "Controller", "Controller Top", "Bleed cover"
